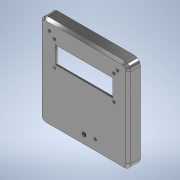
# Autodesk Inventor part: Tampa
Saved by Autodesk Inventor 2021 (Build 250183000, 183)
## iProperties
Created: 2020-12-21
Part Number: Tampa
Material: Generic
Document SubType Name: Modeling
Designer: Vitor
Density: 1 g/cm^3
Appearance: Default
Author: Vitor
Autodesk Inventor part; units mm, degrees
ref_plane "YZ Plane" through (0, 0, 0) normal (1, 0, 0) x (0, 1, 0)
ref_plane "XZ Plane" through (0, 0, 0) normal (0, 1, 0) x (-1, 0, 0)
ref_plane "XY Plane" through (0, 0, 0) normal (0, 0, 1) x (1, 0, 0)
sketch "Sketch1" plane through (0, 0, 0) normal (0, 0, 1) x (1, 0, 0)
  line L0 (0, 103.81) -> (0, 0)
  line L1 (99.04, 103.81) -> (0, 103.81)
  line L2 (99.04, 0) -> (99.04, 103.81)
  circle A0 centre (91.5302, 97.8155) radius 1.6
  circle A1 centre (6.3166, 98.2023) radius 1.6
  circle A2 centre (63.7434, 9.4559) radius 1.6
  line L3 (-2.8877, 39.67) -> (-2.8877, 25.07)
  line L4 (18.04, 39.67) -> (-2.8877, 39.67)
  line L5 (-2.8877, 25.07) -> (18.04, 25.07)
  line L6 (5.99, 20.97) -> (-0.5, 20.97)
  line L7 (-0.5, 20.97) -> (-0.5, 9.286)
  line L8 (-0.5, 9.286) -> (5.99, 9.286)
  line L9 (5.99, 9.286) -> (5.99, 20.97)
  line L10 (18.04, 25.07) -> (18.04, 39.67)
  line L11 (0, 0) -> (99.04, 0)
  line L12 (-2, 105.81) -> (-2, -2)
  line L13 (-2, -2) -> (101.04, -2)
  line L14 (101.04, -2) -> (101.04, 105.81)
  line L15 (101.04, 105.81) -> (-2, 105.81)
  line L16 (-6, 109.81) -> (-6, -6)
  line L17 (-6, -6) -> (105.04, -6)
  line L18 (105.04, -6) -> (105.04, 109.81)
  line L19 (105.04, 109.81) -> (-6, 109.81)
  circle A3 centre (49.53, 7.62) radius 1.55
  point P0 (0, 20.97)
  point P1 (0, 9.286)
  dimension "d0" = 2
  dimension "d1" = 4
  constraints: 40 end point, 4 centre point, 2 horizontal, 2 vertical, 6 other
  measures "d0" distance between parallel lines of L1 L15
  measures "d1" distance between parallel lines of L15 L19
extrude "Extrusion3" add sketch "Sketch1" against normal blind 15 contours L0 L4 L12 L15 L14 L13 L5 L6 L7 L8 L11 L2 L1 | L0 L5 L12 L4 | L12 L5 L3 L4 | L0 L8 L7 L6 | L19 L18 L17 L16
extrude "Extrusion4" add sketch "Sketch1" against normal blind 2 contours L1 L2 L11 L0 L8 L9 L6 L5 L10 L4 | L4 L10 L5 L0 | L6 L9 L8 L0 | A3
fillet "Fillet2" radius 8 4 edges at (105.04, -6, -7.5) (-6, -6, -7.5) (-6, 109.81, -7.5) (105.04, 109.81, -7.5)
chamfer "Chamfer2" distance 3 angle 45 8 edges at (-6, 51.905, 0) (-3.6569, -3.6569, 0) (49.52, -6, 0) (102.6969, -3.6569, 0) (105.04, 51.905, 0) (102.6969, 107.4669, 0) (49.52, 109.81, 0) (-3.6569, 107.4669, 0)
sketch "Sketch2" plane through (0, 0, 0) normal (0, 0, 1) x (1, 0, 0)
  circle A0 centre (49.53, 7.62) radius 1.55 projected
  circle A1 centre (49.53, 7.62) radius 2.5
  point P0 (0, 0)
  dimension "d18" = 5
  constraints: 1 centre point, 1 coincident
  measures "d18" diameter of A1
extrude "Extrusion5" cut sketch "Sketch2" against normal blind 2 contours A0 | A1
sketch "Sketch3" plane through (0, 0, 0) normal (0, 0, 1) x (1, 0, 0)
  line L0 (9.9957, 94.7225) -> (9.9957, 59.1825)
  line L1 (9.9957, 59.1825) -> (90.0757, 59.1825)
  line L2 (90.0757, 59.1825) -> (90.0757, 94.7225)
  line L3 (90.0757, 94.7225) -> (9.9957, 94.7225)
  circle A0 centre (12.6104, 92.4416) radius 1.595
  circle A1 centre (87.094, 61.4588) radius 1.595
  line L4 (13.9957, 86.8134) -> (13.9957, 65.1061)
  line L5 (85.3757, 86.8134) -> (13.9957, 86.8134)
  line L6 (85.3757, 65.1061) -> (85.3757, 86.8134)
  line L7 (13.9957, 65.1061) -> (85.3757, 65.1061)
  circle A2 centre (87.094, 92.4416) radius 1.595
  circle A3 centre (12.6104, 61.4588) radius 1.595
  line L8 (49.6857, 86.8134) -> (49.6857, 75.9598)
  line L9 (2, 106.81) -> (97.04, 106.81) projected
  point P0 (0, 0)
  point P1 (55.3023, 77.61)
  constraints: 18 end point, 4 centre point, 1 midpoint, 1 vertical
extrude "Extrusion6" cut sketch "Sketch3" against normal blind 2 contours A0 | A1 | L5 L6 L7 L4 | A2 | A3
body "Solid2"
